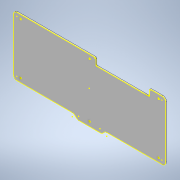
# Autodesk Inventor part: KeyBoardHolder
Saved by Autodesk Inventor 2022 (Build 260153000, 153)
## iProperties
Created: 2021-04-22
Part Number: KeyBoardHolder
Material: Generic
Document SubType Name: Modeling
Designer: Viktor
Density: 1 g/cm^3
Appearance: Default
Author: Viktor
Autodesk Inventor part; units mm, degrees
ref_plane "YZ Plane" through (0, 0, 0) normal (1, 0, 0) x (0, 1, 0)
ref_plane "XZ Plane" through (0, 0, 0) normal (0, 1, 0) x (-1, 0, 0)
ref_plane "XY Plane" through (0, 0, 0) normal (0, 0, 1) x (1, 0, 0)
sketch "Sketch1" plane through (0, 0, 0) normal (0, 0, 1) x (1, 0, 0)
  line L0 (-212.5, -82.5) -> (212.5, -82.5)
  line L1 (212.5, -82.5) -> (212.5, 82.5)
  line L2 (212.5, 82.5) -> (-212.5, 82.5)
  line L3 (-212.5, 82.5) -> (-212.5, -82.5)
  line L4 (-212.5, -82.5) -> (212.5, 82.5) construction
  line L5 (212.5, -82.5) -> (-212.5, 82.5) construction
  line L6 (0, 118.3995) -> (0, -118.3995) construction
  circle A0 centre (0, 71.5) radius 2.25
  circle A1 centre (-192.5, 71.5) radius 2.25
  line L7 (-300.3995, 0) -> (300.3995, 0) projected
  circle A2 centre (192.5, 71.5) radius 2.25
  circle A3 centre (0, -71.5) radius 2.25 construction
  circle A4 centre (-192.5, -71.5) radius 2.25
  circle A5 centre (192.5, -71.5) radius 2.25
  line L8 (-194.25, 0.5) -> (-194.25, -40.0844) construction
  circle A6 centre (0, -79.5) radius 2.25
  point P0 (0, 0)
  dimension "d0" = 425
  dimension "d1" = 165
  dimension "d2" = 4.5
  dimension "d3" = 71.5
  dimension "d4" = 192.5
  dimension "d5" = 4.5
  dimension "d6" = 71.5
  dimension "d12" = 72
  dimension "d14" = 194.25
  dimension "d24" = 8
  dimension "d25" = 4.5
  constraints: 14 end point, 7 centre point, 4 symmetric about line, 2 midpoint, 2 parallel, 2 point on line, 1 horizontal, 1 perpendicular, 1 vertical, 4 other
  measures "d0" distance of L1.end L2.end
  measures "d1" distance of L2.end L0.start
  measures "d2" diameter of A0
  measures "d3" distance of point (0, 0) A0.centre
  measures "d4" distance of A0.centre A1.centre
  measures "d5" diameter of A1
  measures "d6" distance from line of L7 A1.centre
  measures "d12" vertical distance of A4.centre L8.start
  measures "d14" distance from line of L6 L8.start
  measures "d24" distance of A3.centre A6.centre
  measures "d25" diameter of A6
extrude "Extrusion1" add sketch "Sketch1" along normal blind 3
fillet "Fillet1" radius 10 4 edges at (-212.5, -82.5, 1.5) (-212.5, 82.5, 1.5) (212.5, -82.5, 1.5) (212.5, 82.5, 1.5)
sketch "Sketch3" plane through (0, 0, 3) normal (0, 0, 1) x (1, 0, 0)
  line L0 (17.5, 82.5) -> (167.5, 82.5)
  line L1 (167.5, 82.5) -> (167.5, 63.5)
  line L2 (167.5, 63.5) -> (17.5, 63.5)
  line L3 (17.5, 63.5) -> (17.5, 82.5)
  line L4 (202.5, 82.5) -> (-202.5, 82.5) projected
  line L5 (212.5, -72.5) -> (212.5, 72.5) projected
  point P0 (0, 0)
  dimension "d18" = 45
  dimension "d19" = 150
  dimension "d20" = 19
  constraints: 8 end point, 2 parallel, 1 horizontal, 1 perpendicular, 1 point on line
  measures "d18" distance between parallel lines of L5 L1
  measures "d19" distance between parallel lines of L1 L3
  measures "d20" distance of L0.end L1.end
extrude "Extrusion2" cut sketch "Sketch3" against normal blind 3
fillet "Fillet2" radius 2 4 edges at (17.5, 63.5, 1.5) (17.5, 82.5, 1.5) (167.5, 82.5, 1.5) (167.5, 63.5, 1.5)
sketch "Sketch6" plane through (0, 0, 3) normal (0, 0, 1) x (1, 0, 0)
  line L0 (0, 117.5) -> (0, -127.5) projected
  line L1 (-202.5, -82.5) -> (202.5, -82.5) projected
  line L2 (-202.5, -82.5) -> (202.5, -82.5) projected
  line L3 (-44, -82.5) -> (-34, -92.5)
  line L4 (-34, -92.5) -> (0, -92.5)
  line L5 (44, -82.5) -> (34, -92.5)
  line L6 (34, -92.5) -> (0, -92.5)
  point P0 (0, 0)
  dimension "d26" = 45
  dimension "d27" = 10
  constraints: 8 end point, 2 point on line, 2 symmetric about line, 1 perpendicular
  measures "d26" angle of L1 L3
  measures "d27" distance between parallel lines of L1 L4
extrude "Extrusion3" add sketch "Sketch6" against normal up to surface (3 mm away)
fillet "Fillet3" radius 10 4 edges at (-44, -82.5, 1.5) (-34, -92.5, 1.5) (34, -92.5, 1.5) (44, -82.5, 1.5)
sketch "Sketch7" plane through (0, 0, 3) normal (0, 0, 1) x (1, 0, 0)
  circle A0 centre (192.5, 71.5) radius 2.25 projected
  circle A1 centre (-192.5, 71.5) radius 2.25 projected
  circle A2 centre (0, 71.5) radius 2.25 projected
  circle A3 centre (-192.5, -71.5) radius 2.25 projected
  circle A4 centre (192.5, -71.5) radius 2.25 projected
  circle A5 centre (0, -79.5) radius 2.25 projected
  arc A6 (29.8579, -92.5) -> (36.9289, -89.5711) centre (29.8579, -82.5) ccw projected
  line L0 (36.9289, -89.5711) -> (41.0711, -85.4289) projected
  arc A7 (48.1421, -82.5) -> (41.0711, -85.4289) centre (48.1421, -92.5) ccw projected
  line L1 (48.1421, -82.5) -> (202.5, -82.5) projected
  arc A8 (202.5, -82.5) -> (212.5, -72.5) centre (202.5, -72.5) ccw projected
  line L2 (212.5, -72.5) -> (212.5, 72.5) projected
  arc A9 (212.5, 72.5) -> (202.5, 82.5) centre (202.5, 72.5) ccw projected
  line L3 (202.5, 82.5) -> (169.5, 82.5) projected
  arc A10 (169.5, 82.5) -> (167.5, 80.5) centre (169.5, 80.5) ccw projected
  line L4 (167.5, 80.5) -> (167.5, 65.5) projected
  arc A11 (165.5, 63.5) -> (167.5, 65.5) centre (165.5, 65.5) ccw projected
  line L5 (165.5, 63.5) -> (19.5, 63.5) projected
  arc A12 (17.5, 65.5) -> (19.5, 63.5) centre (19.5, 65.5) ccw projected
  line L6 (17.5, 65.5) -> (17.5, 80.5) projected
  arc A13 (17.5, 80.5) -> (15.5, 82.5) centre (15.5, 80.5) ccw projected
  line L7 (15.5, 82.5) -> (-202.5, 82.5) projected
  arc A14 (-202.5, 82.5) -> (-212.5, 72.5) centre (-202.5, 72.5) ccw projected
  line L8 (-212.5, 72.5) -> (-212.5, -72.5) projected
  arc A15 (-212.5, -72.5) -> (-202.5, -82.5) centre (-202.5, -72.5) ccw projected
  line L9 (-202.5, -82.5) -> (-48.1421, -82.5) projected
  arc A16 (-41.0711, -85.4289) -> (-48.1421, -82.5) centre (-48.1421, -92.5) ccw projected
  line L10 (-41.0711, -85.4289) -> (-36.9289, -89.5711) projected
  arc A17 (-36.9289, -89.5711) -> (-29.8579, -92.5) centre (-29.8579, -82.5) ccw projected
  line L11 (-29.8579, -92.5) -> (29.8579, -92.5) projected
  point P0 (0, 0)
equation "\"d5\" = d2"
equation "\"d6\" = d3"
equation "\"d25\" = d5"
body "Solid1"
